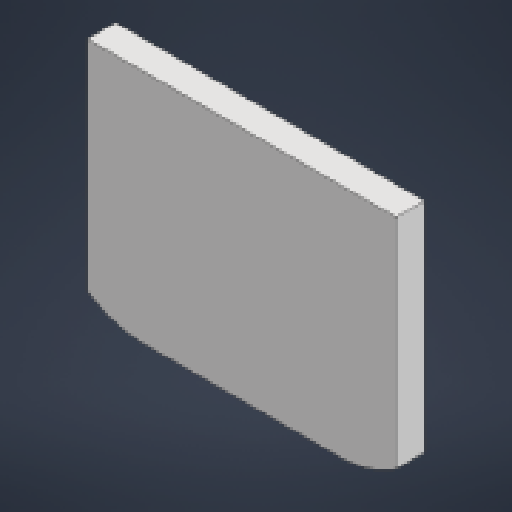
# Autodesk Inventor part: 真键盘外壳
Saved by Autodesk Inventor 2025 (Build 290162000, 162)
## iProperties
Created: 2025-11-30
Part Number: 真键盘外壳
Material: 常规
Document SubType Name: Modeling
Designer: XH
Density: 1 g/cm^3
Appearance: 默认
Author: XH
Autodesk Inventor part; units mm, degrees
ref_plane "YZ Plane" through (0, 0, 0) normal (1, 0, 0) x (0, 1, 0)
ref_plane "XZ Plane" through (0, 0, 0) normal (0, 1, 0) x (-1, 0, 0)
ref_plane "XY Plane" through (0, 0, 0) normal (0, 0, 1) x (1, 0, 0)
sketch "草图1" plane through (0, 0, 0) normal (0, 0, 1) x (1, 0, 0)
  arc A0 (24.3569, -28.6353) -> (34.3569, -25.6353) centre (23.2668, -6.8349) ccw projected
  line L0 (34.3569, -25.6353) -> (34.3569, 23.3647) projected
  line L1 (34.3569, 23.3647) -> (-35.6431, 23.3647) projected
  line L2 (-35.6431, 23.3647) -> (-35.6431, -25.6353) projected
  arc A1 (-35.6431, -25.6353) -> (-25.6431, -28.6353) centre (-24.5529, -6.8349) ccw projected
  line L3 (-25.6431, -28.6353) -> (24.3569, -28.6353) projected
  line L4 (-38.6431, 26.3647) -> (37.3569, 26.3647)
  line L5 (37.3569, 26.3647) -> (37.3569, -27.277)
  arc A2 (24.4295, -31.6353) -> (37.3569, -27.277) centre (23.2668, -6.8349) ccw
  line L6 (24.4295, -31.6353) -> (-25.7156, -31.6353)
  arc A3 (-38.6431, -27.277) -> (-25.7156, -31.6353) centre (-24.5529, -6.8349) ccw
  line L7 (-38.6431, -27.277) -> (-38.6431, 26.3647)
  dimension "d2" = 3
  constraints: 8 end point, 4 point on circle, 2 centre point, 5 other
  measures "d2" distance between parallel lines of L1 L4
extrude "拉伸2" add sketch "草图1" along normal blind 2 contours L3 A1 L2 L1 L0 A0 | L4 L5 A2 L6 A3 L7
sketch "草图2" plane through (0, 0, 0) normal (0, 0, -1) x (-1, 0, 0)
  arc A0 (-34.3569, -25.6353) -> (-24.3569, -28.6353) centre (-23.2668, -6.8349) ccw projected
  line L0 (25.6431, -28.6353) -> (-24.3569, -28.6353) projected
  arc A1 (25.6431, -28.6353) -> (35.6431, -25.6353) centre (24.5529, -6.8349) ccw projected
  line L1 (35.6431, 23.3647) -> (35.6431, -25.6353) projected
  line L2 (-34.3569, 23.3647) -> (35.6431, 23.3647) projected
  line L3 (-34.3569, -25.6353) -> (-34.3569, 23.3647) projected
  arc A2 (25.7156, -31.6353) -> (38.6431, -27.277) centre (24.5529, -6.8349) ccw
  line L4 (25.7156, -31.6353) -> (-24.4295, -31.6353)
  arc A3 (-37.3569, -27.277) -> (-24.4295, -31.6353) centre (-23.2668, -6.8349) ccw
  line L5 (-37.3569, -27.277) -> (-37.3569, 26.3647)
  line L6 (-37.3569, 26.3647) -> (38.6431, 26.3647)
  line L7 (38.6431, 26.3647) -> (38.6431, -27.277)
  point P0 (0, 0)
  dimension "d5" = 3
  constraints: 8 end point, 4 point on circle, 2 centre point, 5 other
  measures "d5" radial gap between concentric circles of A1 A2
extrude "拉伸3" add sketch "草图2" along normal blind 5
